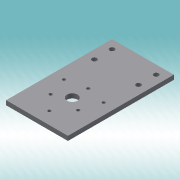
# Autodesk Inventor part: エンコーダ取り付け板
Saved by Autodesk Inventor 2015 (Build 190159000, 159)
## iProperties
Created: 2016-02-19
Part Number: エンコーダ取り付け板
Material: 一般
Document SubType Name: Modeling
Designer: buzztaka
Density: 1 g/cm^3
Appearance: 既定
Author: buzztaka
Autodesk Inventor part; units mm, degrees
ref_plane "YZ Plane" through (0, 0, 0) normal (1, 0, 0) x (0, 1, 0)
ref_plane "XZ Plane" through (0, 0, 0) normal (0, 1, 0) x (-1, 0, 0)
ref_plane "XY Plane" through (0, 0, 0) normal (0, 0, 1) x (1, 0, 0)
sketch "スケッチ1" plane through (0, 0, 0) normal (0, 0, 1) x (1, 0, 0)
  line L0 (0, 0) -> (70, 0)
  line L1 (70, 0) -> (70, 120)
  line L2 (70, 120) -> (0, 120)
  line L3 (0, 120) -> (0, 0)
  dimension "d0" = 70
  dimension "d1" = 120
  constraints: 8 end point, 2 parallel, 1 horizontal, 1 perpendicular
  measures "d0" distance of L0.start L0.end
  measures "d1" distance of L2.end L0.start
extrude "押し出し1" add sketch "スケッチ1" along normal blind 5
sketch "スケッチ2" plane through (0, 0, 5) normal (0, 0, 1) x (1, 0, 0)
  line L0 (0, 120) -> (0, 0) projected
  line L1 (0, 0) -> (70, 0) projected
  point P0 (35, 40)
  dimension "d4" = 35
  dimension "d5" = 40
  measures "d4" distance from line of L0 point (35, 40)
  measures "d5" distance from line of point (35, 40) L1
hole "穴1" at (35, 40, 5) direction (0, 0, -1) diameter 12 end through all
sketch "スケッチ3" plane through (0, 0, 5) normal (0, 0, 1) x (1, 0, 0)
  circle A0 centre (35, 40) radius 6 projected
  point P0 (0, 0)
  point P1 (34.9431, 14)
  point P2 (57.5451, 52.9507)
  point P3 (12.5118, 53.0493)
  dimension "d13" = 26
  dimension "d16" = 360
  constraints: 1 coincident, 4 other
  measures "d13" vertical distance of point (34.943, 14) point (35, 40)
hole "穴2" at (34.9431, 14, 5) at (35, 40, 5) at (57.5451, 52.9507, 5) at (12.5118, 53.0493, 5) direction (0, 0, -1) diameter 3.5 end through all
sketch "スケッチ4" plane through (0, 0, 5) normal (0, 0, 1) x (1, 0, 0)
  line L0 (0, 120) -> (0, 0) projected
  line L1 (0, 0) -> (70, 0) projected
  point P0 (35, 40)
  point P1 (35, 58)
  point P2 (19.4115, 31)
  point P3 (50.5885, 31)
  dimension "d27" = 35
  dimension "d28" = 40
  dimension "d29" = 18
  dimension "d32" = 360
  constraints: 4 other
  measures "d27" distance from line of L0 point (35, 40)
  measures "d28" distance from line of L1 point (35, 40)
  measures "d29" distance of point (35, 58) point (35, 40)
hole "穴3" at (35, 40, 5) at (35, 58, 5) at (19.4115, 31, 5) at (50.5885, 31, 5) direction (0, 0, -1) diameter 3.5 end through all
sketch "スケッチ6" plane through (0, 0, 5) normal (0, 0, 1) x (1, 0, 0)
  line L0 (0, 120) -> (0, 0) projected
  line L1 (0, 0) -> (70, 0) projected
  point P0 (35, 40)
  point P1 (10, 110)
  point P2 (60, 110)
  point P3 (10, 90)
  point P4 (60, 90)
  dimension "d43" = 35
  dimension "d44" = 40
  dimension "d48" = 110
  dimension "d49" = 110
  dimension "d50" = 90
  dimension "d51" = 90
  measures "d43" distance from line of point (35, 40) L0
  measures "d44" distance from line of L1 point (35, 40)
  measures "d48" distance from line of L1 point (10, 110)
  measures "d49" distance from line of L1 point (60, 110)
  measures "d50" distance from line of L1 point (60, 90)
  measures "d51" distance from line of L1 point (10, 90)
hole "穴4" at (35, 40, 5) at (10, 110, 5) at (60, 110, 5) at (10, 90, 5) at (60, 90, 5) direction (0, 0, -1) diameter 5.5 end through all
